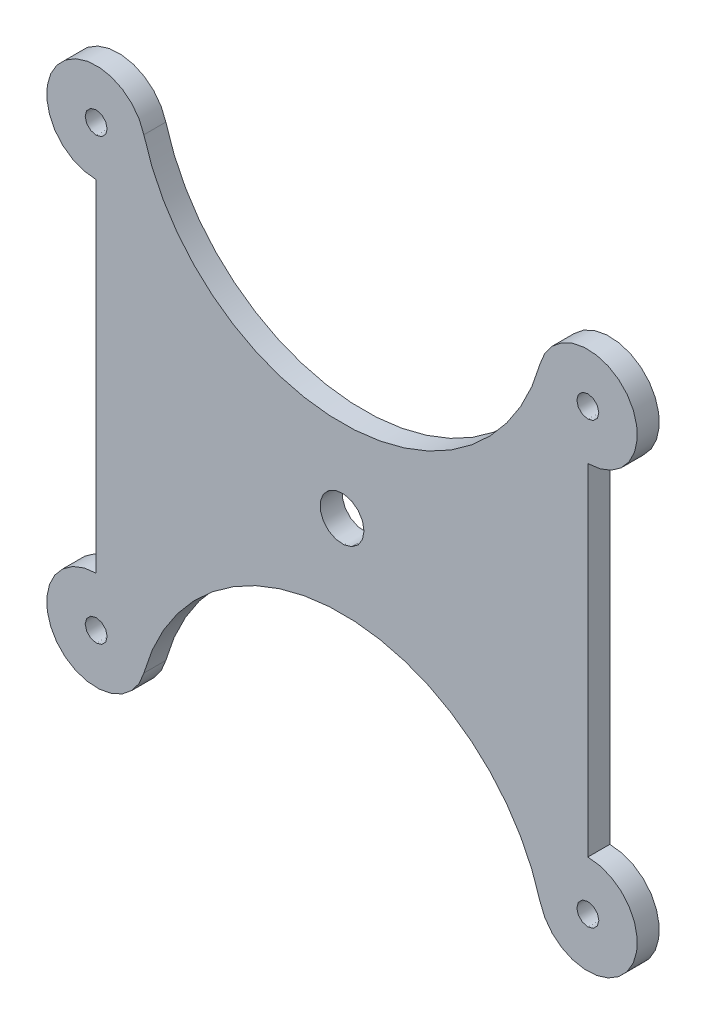
# Autodesk Inventor part: protector carrete
Saved by Autodesk Inventor 2017 (Build 210142000, 142)
## iProperties
Part Number: protector carrete
Material: Genérico
Document SubType Name: Modeling
Designer: FABLAB
Density: 1 g/cm^3
Appearance: Valor por defecto
Author: FABLAB
Autodesk Inventor part; units mm, degrees
ref_plane "YZ Plane" through (0, 0, 0) normal (1, 0, 0) x (0, 1, 0)
ref_plane "XZ Plane" through (0, 0, 0) normal (0, 1, 0) x (-1, 0, 0)
ref_plane "XY Plane" through (0, 0, 0) normal (0, 0, 1) x (1, 0, 0)
sketch "Boceto1" plane through (0, 0, 0) normal (0, 0, 1) x (1, 0, 0)
  circle A0 centre (27.2786, 40) radius 2 projected
  circle A1 centre (116.7214, 40) radius 2 projected
  circle A2 centre (116.7214, -40) radius 2 projected
  circle A3 centre (27.2786, -40) radius 2 projected
  circle A4 centre (72, 0) radius 4 projected
  arc A5 (35.9508, 42.4068) -> (27.2786, 31) centre (27.2786, 40) ccw
  arc A6 (35.9508, 42.4068) -> (108.0492, 42.4068) centre (72, 52.4118) ccw
  arc A7 (116.7214, 31) -> (108.0492, 42.4068) centre (116.7214, 40) ccw
  line L0 (116.7214, 31) -> (116.7214, -31)
  arc A8 (108.0492, -42.4068) -> (116.7214, -31) centre (116.7214, -40) ccw
  arc A9 (108.0492, -42.4068) -> (35.9508, -42.4068) centre (72, -52.4118) ccw
  arc A10 (27.2786, -31) -> (35.9508, -42.4068) centre (27.2786, -40) ccw
  line L1 (27.2786, -31) -> (27.2786, 31)
  circle A11 centre (72, 0) radius 15 construction
  point P0 (0, 0)
  dimension "d0" = 9
  dimension "d1" = 30
  constraints: 12 point on circle, 7 centre point, 6 tangent, 4 concentric, 4 end point, 3 equal radius, 2 point on line, 2 vertical, 1 coincident
  measures "d0" radius of A5
  measures "d1" diameter of A11
extrude "Extrusión1" add sketch "Boceto1" along normal blind 4
